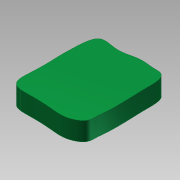
# Autodesk Inventor part: SOIC-08 board
Saved by Autodesk Inventor 2011 (Build 150239000, 239)
## iProperties
Created: 2010-12-28
Part Number: SOIC-08 board
Document SubType Name: Modeling
Designer: abbath
Density: 1 g/cm^3
Author: abbath
Autodesk Inventor part; units mm, degrees
ref_plane "YZ Plane" through (0, 0, 0) normal (1, 0, 0) x (0, 1, 0)
ref_plane "XZ Plane" through (0, 0, 0) normal (0, 1, 0) x (-1, 0, 0)
ref_plane "XY Plane" through (0, 0, 0) normal (0, 0, 1) x (1, 0, 0)
ref_plane "РабПлоскость3" through (0, 0, 0) normal (0, 0, 1) x (1, 0, 0)
sketch "Эскиз4" plane through (0, 0, 0) normal (0, 0, 1) x (1, 0, 0)
  spline S0 degree 5 poles (-0.2383, -0.3169) (0.0455, -0.353) (0.5759, -0.3379) (1.4607, -0.2741) (3.0577, -0.5121) (3.6122, -0.4869) (4.9851, 0.0458) (4.5852, 0.886) (4.9186, 1.2787) (4.7801, 4.3212) (4.7337, 4.7475) (4.864, 6.5266) (4.0123, 6.6387) (3.6249, 6.4612) (2.2527, 6.9221) (1.1797, 6.0216) (-0.5021, 6.879) (-0.8333, 6.2027) (-0.9921, 5.5473) (-0.9799, 4.4715) (-1.0698, 3.6135) (-0.8339, 1.6898) (-1.2107, 0.2625) (-0.8562, -0.1698) (-0.4883, -0.285) (-0.2383, -0.3169) knots 0 0 0 0 0 0 0.067521 0.108633 0.15626 0.200019 0.24646 0.295244 0.344851 0.394055 0.442121 0.484598 0.528138 0.573068 0.618175 0.664068 0.708834 0.751105 0.796603 0.846872 0.897913 0.940501 1 1 1 1 1 1
  point P0 (0, 0)
  point P1 (3.033, -0.4579)
  point P2 (3.9261, -0.3169)
  point P3 (4.6217, 0.1719)
  point P4 (4.7345, 0.6514)
  point P5 (4.7721, 1.2812)
  point P6 (4.7909, 3.9509)
  point P7 (4.7627, 5.3985)
  point P8 (4.4995, 6.3856)
  point P9 (4.1047, 6.5642)
  point P10 (3.6535, 6.5736)
  point P11 (2.5912, 6.6488)
  point P12 (0.871, 6.4138)
  point P13 (-0.4733, 6.4984)
  point P14 (-0.7929, 6.1694)
  point P15 (-0.9339, 5.6147)
  point P16 (-0.9903, 4.7875)
  point P17 (-1.0091, 3.6877)
  point P18 (-0.9997, 1.4128)
  point P19 (-0.8681, 0)
  constraints: 21 other
extrude "Выдавливание4" add sketch "Эскиз4" along normal blind 1.5
